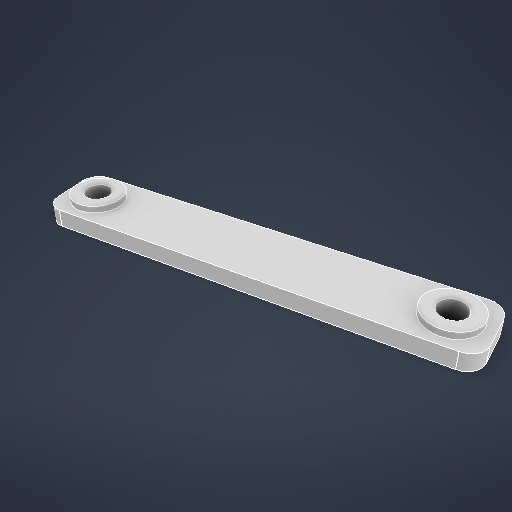
# Autodesk Inventor part: Servo_Steering_Linkage
Saved by Autodesk Inventor 2025 (Build 290162000, 162)
## iProperties
Created: 2024-06-02
Part Number: Servo_Steering_Linkage
Material: Generic
Document SubType Name: Modeling
Designer: chaya
Density: 1 g/cm^3
Appearance: Default
Author: chaya
Autodesk Inventor part; units mm, degrees
ref_plane "YZ Plane" through (0, 0, 0) normal (1, 0, 0) x (0, 1, 0)
ref_plane "XZ Plane" through (0, 0, 0) normal (0, 1, 0) x (-1, 0, 0)
ref_plane "XY Plane" through (0, 0, 0) normal (0, 0, 1) x (1, 0, 0)
derived "Car_Plan.ipt"
sketch "Car_Sketch" plane through (0, 0, 0) normal (0, 1, 0) x (-1, 0, 0)
  line L0 (0, 0) -> (94, 0)
  line L1 (0, 0) -> (0, 105)
  line L2 (94, 0) -> (94, 105)
  line L3 (0, 105) -> (20, 105)
  line L4 (20, 105) -> (20, 190)
  line L5 (20, 190) -> (74, 190)
  line L6 (74, 190) -> (74, 105)
  line L7 (74, 105) -> (94, 105)
  line L8 (-5, 68) -> (-5, 0)
  line L9 (-5, 0) -> (-32, 0)
  line L10 (-32, 0) -> (-32, 68)
  line L11 (-32, 68) -> (-5, 68)
  line L12 (47, 190) -> (47, 0) construction
  line L13 (126, 68) -> (99, 68)
  line L14 (99, 68) -> (99, 0)
  line L15 (126, 0) -> (126, 68)
  line L16 (99, 0) -> (126, 0)
  line L17 (-5, 34) -> (99, 34) construction
  line L18 (0, 95) -> (94, 95) construction
  line L19 (-5, 190) -> (-32, 190)
  line L20 (-32, 122) -> (-5, 122)
  line L21 (-32, 190) -> (-32, 122)
  line L22 (-5, 122) -> (-5, 190)
  line L23 (-5, 156) -> (99, 156) construction
  line L24 (126, 122) -> (99, 122)
  line L25 (126, 190) -> (126, 122)
  line L26 (99, 190) -> (126, 190)
  line L27 (99, 122) -> (99, 190)
  line L28 (0, 156) -> (47, 34) construction
  line L29 (94, 156) -> (47, 34) construction
  line L30 (0, 156) -> (-174.2341, 34) construction
  line L31 (-5, 34) -> (-174.2341, 34) construction
  line L32 (8.9873, 132.6713) -> (47, 142.55) construction
  line L33 (85.0127, 132.6713) -> (47, 142.55) construction
sketch "Base" plane through (0, 0, 0) normal (0, 1, 0) x (-1, 0, 0)
  line L0 (8.9873, 132.6713) -> (47, 142.55) construction
  line L1 (6.122, 127.7938) -> (51.8775, 139.6847)
  line L2 (51.8775, 139.6847) -> (49.8653, 147.4275)
  line L3 (49.8653, 147.4275) -> (4.1098, 135.5366)
  line L4 (4.1098, 135.5366) -> (6.122, 127.7938)
  line L5 (8.9873, 132.6713) -> (7.9812, 136.5427) construction
  line L6 (8.9873, 132.6713) -> (9.9934, 128.7999) construction
  circle A0 centre (8.9873, 132.6713) radius 1.5
  circle A1 centre (47, 142.55) radius 1.5
  point P0 (0, 0)
  dimension "d2" = 8
  dimension "d3" = 4
  dimension "d4" = 4
  dimension "d5" = 3
  dimension "d6" = 3
  constraints: 12 end point, 4 perpendicular, 2 centre point, 2 coincident, 2 collinear, 2 point on line, 1 parallel
  measures "d2" distance of L1.start L3.end
  measures "d3" distance from line of L4 L0.start
  measures "d4" distance from line of L2 L0.end
  measures "d5" diameter of A0
  measures "d6" diameter of A1
extrude "Base_Extrusion" add sketch "Base" along normal blind 2
sketch "Sketch5" plane through (0, 2, 0) normal (0, 1, 0) x (1, 0, 0)
  circle A0 centre (-47, -142.55) radius 1.5 projected
  circle A1 centre (-8.9873, -132.6713) radius 1.5 projected
  circle A2 centre (-47, -142.55) radius 3
  circle A3 centre (-8.9873, -132.6713) radius 1.5 projected
  circle A4 centre (-8.9873, -132.6713) radius 3
  point P0 (0, 0)
  dimension "d18" = 6
  dimension "d19" = 6
  constraints: 2 centre point, 2 coincident
  measures "d18" diameter of A2
  measures "d19" diameter of A4
extrude "Extrusion3" add sketch "Sketch5" along normal blind 0.8
fillet "Fillet1" radius 2 4 edges at (-49.8653, 1, 147.4275) (-51.8775, 1, 139.6847) (-4.1098, 1, 135.5366) (-6.122, 1, 127.7938)
equation "\"d4\" = d3"
body "Solid1"
